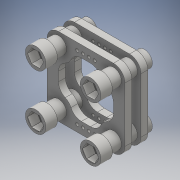
# Autodesk Inventor part: P8X32A_FT232RL_TestJig
Saved by Autodesk Inventor 2016 (Build 200138000, 138)
## iProperties
Created: 2026-06-10
Part Number: P8X32A_FT232RL_TestJig
Material: Generic
Document SubType Name: Modeling
Designer: Steve
Density: 1 g/cm^3
Appearance: Default
Author: Steve
Autodesk Inventor part; units mm, degrees
ref_plane "YZ Plane" through (0, 0, 0) normal (1, 0, 0) x (0, 1, 0)
ref_plane "XZ Plane" through (0, 0, 0) normal (0, 1, 0) x (-1, 0, 0)
ref_plane "XY Plane" through (0, 0, 0) normal (0, 0, 1) x (1, 0, 0)
sketch "Sketch1" plane through (0, 0, 0) normal (0, 1, 0) x (-1, 0, 0)
  line L0 (19.415789, 13.28113) -> (-14.584211, 13.28113)
  line L1 (-14.584211, 13.28113) -> (-14.584211, -20.71887)
  line L2 (-14.584211, -20.71887) -> (19.415789, -20.71887)
  line L3 (19.415789, -20.71887) -> (19.415789, 13.28113)
  circle A0 centre (14.415789, 8.28113) radius 1.75
  circle A1 centre (14.415789, -15.71887) radius 1.75
  circle A2 centre (-9.584211, -15.71887) radius 1.75
  circle A3 centre (-9.584211, 8.28113) radius 1.75
  circle A4 centre (6.215789, 10.28113) radius 0.65
  circle A5 centre (3.675789, 10.28113) radius 0.65
  circle A6 centre (1.135789, 10.28113) radius 0.65
  circle A7 centre (-1.404211, 10.28113) radius 0.65
  circle A8 centre (6.215789, -17.71887) radius 0.65
  circle A9 centre (3.675789, -17.71887) radius 0.65
  circle A10 centre (1.135789, -17.71887) radius 0.65
  circle A11 centre (-1.404211, -17.71887) radius 0.65
  circle A12 centre (14.415789, 8.28113) radius 3.5
  circle A13 centre (14.415789, -15.71887) radius 3.5
  circle A14 centre (-9.584211, -15.71887) radius 3.5
  circle A15 centre (-9.584211, 8.28113) radius 3.5
  line L4 (14.415789, 3.28113) -> (9.415789, 3.28113)
  line L5 (9.415789, 3.28113) -> (9.415789, 8.28113)
  line L6 (9.415789, 8.28113) -> (-4.584211, 8.28113)
  line L7 (-4.584211, 8.28113) -> (-4.584211, 3.28113)
  line L8 (-4.584211, 3.28113) -> (-9.584211, 3.28113)
  line L9 (-9.584211, 3.28113) -> (-9.584211, -10.71887)
  line L10 (-9.584211, -10.71887) -> (-4.584211, -10.71887)
  line L11 (-4.584211, -10.71887) -> (-4.584211, -15.71887)
  line L12 (-4.584211, -15.71887) -> (9.415789, -15.71887)
  line L13 (9.415789, -15.71887) -> (9.415789, -10.71887)
  line L14 (9.415789, -10.71887) -> (14.415789, -10.71887)
  line L15 (14.415789, -10.71887) -> (14.415789, 3.28113)
  point P0 (0, 0)
  dimension "d0" = 34
  dimension "d1" = 34
  dimension "d2" = 3.5
  dimension "d3" = 3.5
  dimension "d4" = 3.5
  dimension "d5" = 3.5
  dimension "d6" = 5
  dimension "d7" = 5
  dimension "d8" = 5
  dimension "d9" = 5
  dimension "d10" = 5
  dimension "d11" = 5
  dimension "d12" = 5
  dimension "d13" = 5
  dimension "d14" = 1.3
  dimension "d15" = 1.3
  dimension "d16" = 1.3
  dimension "d17" = 1.3
  dimension "d18" = 2.54
  dimension "d19" = 3
  dimension "d20" = 2.54
  dimension "d21" = 3
  dimension "d22" = 3
  dimension "d23" = 3
  dimension "d24" = 2.54
  dimension "d25" = 13.2
  dimension "d26" = 1.3
  dimension "d27" = 1.3
  dimension "d28" = 1.3
  dimension "d29" = 1.3
  dimension "d30" = 2.54
  dimension "d31" = 2.54
  dimension "d32" = 2.54
  dimension "d33" = 3
  dimension "d34" = 3
  dimension "d35" = 3
  dimension "d36" = 3
  dimension "d37" = 13.2
  dimension "d38" = 7
  dimension "d39" = 7
  dimension "d40" = 7
  dimension "d41" = 7
  dimension "d42" = 5
  dimension "d43" = 5
  dimension "d44" = 5
  dimension "d45" = 5
  dimension "d46" = 5
  dimension "d47" = 5
  dimension "d48" = 5
  dimension "d49" = 5
  constraints: 32 end point, 16 centre point, 8 perpendicular, 8 point on line, 4 coincident, 2 horizontal, 2 parallel
  measures "d0" distance of L2.end L0.start
  measures "d1" distance of L1.end L2.end
  measures "d2" diameter of A0
  measures "d3" diameter of A1
  measures "d4" diameter of A2
  measures "d5" diameter of A3
  measures "d6" distance from line of L0 A0.centre
  measures "d7" distance from line of L3 A0.centre
  measures "d8" distance from line of L3 A1.centre
  measures "d9" distance from line of L2 A1.centre
  measures "d10" distance from line of L1 A2.centre
  measures "d11" distance from line of L2 A2.centre
  measures "d12" distance from line of L1 A3.centre
  measures "d13" distance from line of L0 A3.centre
  measures "d14" diameter of A4
  measures "d15" diameter of A5
  measures "d16" diameter of A6
  measures "d17" diameter of A7
  measures "d18" distance of A5.centre A4.centre
  measures "d19" distance from line of L0 A4.centre
  measures "d20" distance of A5.centre A6.centre
  measures "d21" distance from line of L0 A5.centre
  measures "d22" distance from line of L0 A6.centre
  measures "d23" distance from line of L0 A7.centre
  measures "d24" distance of A6.centre A7.centre
  measures "d25" distance from line of L3 A4.centre
  measures "d26" diameter of A8
  measures "d27" diameter of A9
  measures "d28" diameter of A10
  measures "d29" diameter of A11
  measures "d30" distance of A9.centre A8.centre
  measures "d31" distance of A10.centre A9.centre
  measures "d32" distance of A10.centre A11.centre
  measures "d33" distance from line of L2 A11.centre
  measures "d34" distance from line of L2 A10.centre
  measures "d35" distance from line of L2 A9.centre
  measures "d36" distance from line of L2 A8.centre
  measures "d37" distance from line of L3 A8.centre
  measures "d38" diameter of A12
  measures "d39" diameter of A13
  measures "d40" diameter of A14
  measures "d41" diameter of A15
  measures "d42" distance between parallel lines of L3 L15
  measures "d43" distance between parallel lines of L9 L1
  measures "d44" distance of L7.end L8.end
  measures "d45" distance of L6.end L7.end
  measures "d46" distance of L13.end L14.end
  measures "d47" distance between parallel lines of L0 L6
  measures "d48" distance between parallel lines of L2 L12
  measures "d49" distance of L10.end L11.end
sketch "Sketch1 outline for Extrusion1" plane through (0, 0, 0) normal (0, 1, 0) x (-1, 0, 0)
  line L0 (19.415789, -20.71887) -> (19.415789, 13.28113)
  line L1 (-14.584211, -20.71887) -> (19.415789, -20.71887)
  line L2 (19.415789, 13.28113) -> (-14.584211, 13.28113)
  line L3 (-14.584211, 13.28113) -> (-14.584211, -20.71887)
  circle A0 centre (-9.584211, -15.71887) radius 3.5
  circle A1 centre (-1.404211, -17.71887) radius 0.65
  circle A2 centre (1.135789, -17.71887) radius 0.65
  circle A3 centre (3.675789, -17.71887) radius 0.65
  circle A4 centre (6.215789, -17.71887) radius 0.65
  circle A5 centre (14.415789, -15.71887) radius 3.5
  circle A6 centre (-9.584211, 8.28113) radius 3.5
  circle A7 centre (-1.404211, 10.28113) radius 0.65
  circle A8 centre (1.135789, 10.28113) radius 0.65
  line L4 (14.415789, -10.71887) -> (14.415789, 3.28113)
  line L5 (14.415789, 3.28113) -> (9.415789, 3.28113)
  line L6 (9.415789, 3.28113) -> (9.415789, 8.28113)
  line L7 (9.415789, 8.28113) -> (-4.584211, 8.28113)
  line L8 (-4.584211, 8.28113) -> (-4.584211, 3.28113)
  line L9 (-4.584211, 3.28113) -> (-9.584211, 3.28113)
  line L10 (-9.584211, 3.28113) -> (-9.584211, -10.71887)
  line L11 (-9.584211, -10.71887) -> (-4.584211, -10.71887)
  line L12 (-4.584211, -10.71887) -> (-4.584211, -15.71887)
  line L13 (-4.584211, -15.71887) -> (9.415789, -15.71887)
  line L14 (9.415789, -15.71887) -> (9.415789, -10.71887)
  line L15 (9.415789, -10.71887) -> (14.415789, -10.71887)
  circle A9 centre (3.675789, 10.28113) radius 0.65
  circle A10 centre (6.215789, 10.28113) radius 0.65
  circle A11 centre (14.415789, 8.28113) radius 3.5
extrude "Extrusion1" add sketch "Sketch1 outline for Extrusion1" against normal blind 10
fillet "Fillet1" radius 5 16 edges at (-9.4158, -5, -10.7189) (4.5842, -5, -10.7189) (4.5842, -5, 3.2811) (-9.4158, -5, 3.2811) (-14.4158, -5, 3.2811) (-14.4158, -5, -10.7189) (-9.4158, -5, -15.7189) (4.5842, -5, -15.7189) (9.5842, -5, -10.7189) (9.5842, -5, 3.2811) (4.5842, -5, 8.2811) (-9.4158, -5, 8.2811) (14.5842, -5, 13.2811) (-19.4158, -5, 13.2811) (-19.4158, -5, -20.7189) (14.5842, -5, -20.7189)
sketch "Sketch1 outline for Extrusion2" plane through (0, 0, 0) normal (0, 1, 0) x (-1, 0, 0)
  circle A0 centre (14.415789, 8.28113) radius 3.5
  circle A1 centre (14.415789, 8.28113) radius 1.75
  circle A2 centre (14.415789, -15.71887) radius 3.5
  circle A3 centre (14.415789, -15.71887) radius 1.75
  circle A4 centre (-9.584211, -15.71887) radius 3.5
  circle A5 centre (-9.584211, -15.71887) radius 1.75
  circle A6 centre (-9.584211, 8.28113) radius 3.5
  circle A7 centre (-9.584211, 8.28113) radius 1.75
extrude "Extrusion2" add sketch "Sketch1 outline for Extrusion2" against normal blind 10
sketch "Sketch2" plane through (-14.415789, 0, 13.28113) normal (0, 0, 1) x (1, 0, 0)
  line L0 (-5, -3) -> (29, -3)
  line L1 (29, -3) -> (29, -7)
  line L2 (29, -7) -> (-5, -7)
  line L3 (-5, -7) -> (-5, -3)
  line L4 (29, -10) -> (29, 0) projected
  line L5 (-5, 0) -> (-5, -10) projected
  line L6 (0, 0) -> (24, 0) projected
  line L7 (24, -10) -> (0, -10) projected
  point P0 (14.415789, 0)
  dimension "d59" = 0
  dimension "d60" = 0
  dimension "d61" = 3
  dimension "d62" = 3
  constraints: 8 end point, 2 parallel, 1 horizontal, 1 perpendicular
  measures "d59" distance between parallel lines of L4 L1
  measures "d60" distance between parallel lines of L5 L3
  measures "d61" distance between parallel lines of L6 L0
  measures "d62" distance between parallel lines of L7 L2
sketch "Sketch2 outline for Extrusion5" plane through (-14.415789, 0, 13.28113) normal (0, 0, 1) x (1, 0, 0)
  line L0 (-5, -3) -> (29, -3)
  line L1 (29, -3) -> (29, -7)
  line L2 (29, -7) -> (-5, -7)
  line L3 (-5, -7) -> (-5, -3)
extrude "Extrusion5" cut sketch "Sketch2 outline for Extrusion5" against normal through all
sketch "Sketch1 outline for Extrusion3" plane through (0, 0, 0) normal (0, 1, 0) x (-1, 0, 0)
  circle A0 centre (14.415789, 8.28113) radius 3.5
  circle A1 centre (14.415789, 8.28113) radius 1.75
  circle A2 centre (14.415789, -15.71887) radius 3.5
  circle A3 centre (14.415789, -15.71887) radius 1.75
  circle A4 centre (-9.584211, -15.71887) radius 3.5
  circle A5 centre (-9.584211, -15.71887) radius 1.75
  circle A6 centre (-9.584211, 8.28113) radius 3.5
  circle A7 centre (-9.584211, 8.28113) radius 1.75
extrude "Extrusion3" add sketch "Sketch1 outline for Extrusion3" along normal blind 3.5
sketch "Sketch1 outline for Extrusion4" plane through (0, 0, 0) normal (0, 1, 0) x (-1, 0, 0)
  circle A0 centre (14.415789, 8.28113) radius 3.5
  circle A1 centre (14.415789, 8.28113) radius 1.75
  circle A2 centre (14.415789, -15.71887) radius 3.5
  circle A3 centre (14.415789, -15.71887) radius 1.75
  circle A4 centre (-9.584211, -15.71887) radius 3.5
  circle A5 centre (-9.584211, -15.71887) radius 1.75
  circle A6 centre (-9.584211, 8.28113) radius 3.5
  circle A7 centre (-9.584211, 8.28113) radius 1.75
extrude "Extrusion4" add sketch "Sketch1 outline for Extrusion4" against normal blind 20
sketch "Sketch3" plane through (9.584211, -20, 8.28113) normal (0, -1, 0) x (1, 0, 0)
  circle A0 centre (0, 0) radius 3.5
  circle A1 centre (0, 0) radius 4.5
  circle A2 centre (0, -24.009901) radius 3.5
  circle A3 centre (0, -24.009901) radius 4.5
  circle A4 centre (-24, -24.009901) radius 3.5
  circle A5 centre (-24, -24.009901) radius 4.5
  circle A6 centre (-24, 0) radius 3.5
  circle A7 centre (-24, 0) radius 4.5
  circle A8 centre (0, -24) radius 3.5
  line L0 (3.499996, -24.004951) -> (1.754286, -27.038512)
  line L1 (1.754286, -27.038512) -> (-1.745711, -27.043463)
  line L2 (-1.745711, -27.043463) -> (-3.499996, -24.014852)
  line L3 (-3.499996, -24.014852) -> (-1.754286, -20.981291)
  line L4 (-1.754286, -20.981291) -> (1.745711, -20.97634)
  line L5 (1.745711, -20.97634) -> (3.499996, -24.004951)
  circle A9 centre (-24, -24) radius 3.5
  line L6 (-20.500004, -24.004951) -> (-22.245714, -27.038512)
  line L7 (-22.245714, -27.038512) -> (-25.745711, -27.043463)
  line L8 (-25.745711, -27.043463) -> (-27.499996, -24.014852)
  line L9 (-27.499996, -24.014852) -> (-25.754286, -20.981291)
  line L10 (-25.754286, -20.981291) -> (-22.254289, -20.97634)
  line L11 (-22.254289, -20.97634) -> (-20.500004, -24.004951)
  circle A10 centre (0, 0) radius 3.5
  line L12 (3.499999, 0.002005) -> (1.751736, -3.030086)
  line L13 (1.751736, -3.030086) -> (-1.748264, -3.032091)
  line L14 (-1.748264, -3.032091) -> (-3.499999, -0.002005)
  line L15 (-3.499999, -0.002005) -> (-1.751736, 3.030086)
  line L16 (-1.751736, 3.030086) -> (1.748264, 3.032091)
  line L17 (1.748264, 3.032091) -> (3.499999, 0.002005)
  circle A11 centre (-24, 0) radius 3.5
  line L18 (-22.249305, -3.030688) -> (-25.749305, -3.03149)
  line L19 (-25.749305, -3.03149) -> (-27.5, -0.000802)
  line L20 (-27.5, -0.000802) -> (-25.750695, 3.030688)
  line L21 (-25.750695, 3.030688) -> (-22.250695, 3.03149)
  line L22 (-22.250695, 3.03149) -> (-20.5, 0.000802)
  line L23 (-20.5, 0.000802) -> (-22.249305, -3.030688)
  point P0 (-9.584211, -8.28113)
  dimension "d67" = 7
  dimension "d69" = 7
  dimension "d71" = 7
  dimension "d73" = 7
  dimension "d68" = 9
  dimension "d70" = 9
  dimension "d72" = 9
  dimension "d74" = 9
  constraints: 48 end point, 8 coincident, 4 centre point, 72 other
  measures "d68" diameter of A1
  measures "d70" diameter of A3
  measures "d72" diameter of A5
  measures "d74" diameter of A7
sketch "Sketch3 outline for Extrusion6" plane through (9.584211, -20, 8.28113) normal (0, -1, 0) x (1, 0, 0)
  circle A0 centre (0, 0) radius 4.5
  circle A1 centre (0, 0) radius 3.5
  circle A2 centre (0, -24.009901) radius 4.5
  arc A3 (-3.499996, -24.004951) -> (3.499986, -24.009901) centre (0, -24) cw
  arc A4 (-3.499996, -24.004951) -> (3.5, -24.009901) centre (0, -24.009901) ccw
  circle A5 centre (-24, -24.009901) radius 4.5
  arc A6 (-27.499996, -24.004951) -> (-20.500014, -24.009901) centre (-24, -24) cw
  arc A7 (-27.499996, -24.004951) -> (-20.5, -24.009901) centre (-24, -24.009901) ccw
  circle A8 centre (-24, 0) radius 4.5
  circle A9 centre (-24, 0) radius 3.5
extrude "Extrusion6" add sketch "Sketch3 outline for Extrusion6" against normal blind 5
sketch "Sketch3 outline for Extrusion7" plane through (9.584211, -20, 8.28113) normal (0, -1, 0) x (1, 0, 0)
  line L0 (3.499999, 0.002005) -> (1.751736, -3.030086)
  line L1 (1.751736, -3.030086) -> (-1.748264, -3.032091)
  line L2 (-1.748264, -3.032091) -> (-3.499999, -0.002005)
  line L3 (-3.499999, -0.002005) -> (-1.751736, 3.030086)
  line L4 (-1.751736, 3.030086) -> (1.748264, 3.032091)
  line L5 (1.748264, 3.032091) -> (3.499999, 0.002005)
  line L6 (3.499996, -24.004951) -> (1.754286, -27.038512)
  line L7 (1.754286, -27.038512) -> (-1.745711, -27.043463)
  line L8 (-1.745711, -27.043463) -> (-3.499996, -24.014852)
  line L9 (-3.499996, -24.014852) -> (-1.754286, -20.981291)
  line L10 (-1.754286, -20.981291) -> (1.745711, -20.97634)
  line L11 (1.745711, -20.97634) -> (3.499996, -24.004951)
  line L12 (-20.500004, -24.004951) -> (-22.245714, -27.038512)
  line L13 (-22.245714, -27.038512) -> (-25.745711, -27.043463)
  line L14 (-25.745711, -27.043463) -> (-27.499996, -24.014852)
  line L15 (-27.499996, -24.014852) -> (-25.754286, -20.981291)
  line L16 (-25.754286, -20.981291) -> (-22.254289, -20.97634)
  line L17 (-22.254289, -20.97634) -> (-20.500004, -24.004951)
  line L18 (-22.249305, -3.030688) -> (-25.749305, -3.03149)
  line L19 (-25.749305, -3.03149) -> (-27.5, -0.000802)
  line L20 (-27.5, -0.000802) -> (-25.750695, 3.030688)
  line L21 (-25.750695, 3.030688) -> (-22.250695, 3.03149)
  line L22 (-22.250695, 3.03149) -> (-20.5, 0.000802)
  line L23 (-20.5, 0.000802) -> (-22.249305, -3.030688)
extrude "Extrusion7" cut sketch "Sketch3 outline for Extrusion7" against normal blind 4
body "Solid1"
